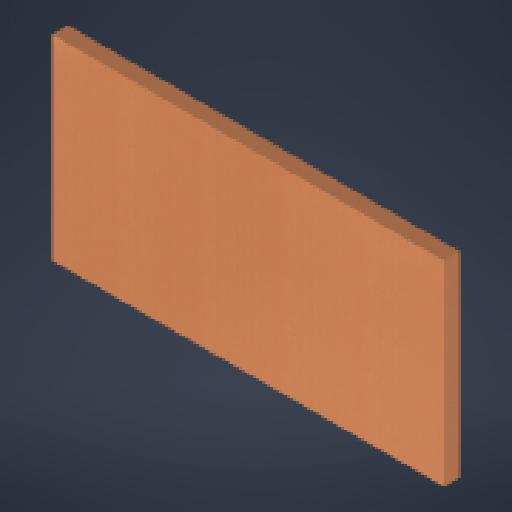
# Autodesk Inventor part: block_of_wood
Saved by Autodesk Inventor 2026 (Build 300175000, 175)
## iProperties
Created: 2025-03-30
Part Number: block_of_wood
Material: Wood (Walnut)
Document SubType Name: Modeling
Designer: paris
Density: 0.55 g/cm^3
Appearance: Walnut - Natural Polished
Author: paris
Autodesk Inventor part; units mm, degrees
ref_plane "YZ Plane" through (0, 0, 0) normal (1, 0, 0) x (0, 1, 0)
ref_plane "XZ Plane" through (0, 0, 0) normal (0, 1, 0) x (-1, 0, 0)
sketch "Sketch1" plane through (0, 0, 0) normal (0, 0, 1) x (1, 0, 0)
  line L0 (25, 1.485) -> (-25, 1.485) projected
  line L1 (0, 1.485) -> (-609.6, 1.485)
  line L2 (-609.6, 1.485) -> (-609.6, 611.085)
  line L3 (-609.6, 611.085) -> (0, 611.085)
  line L4 (0, 611.085) -> (0, 1.485)
  line L5 (0, 611.085) -> (609.6, 611.085)
  line L6 (609.6, 611.085) -> (609.6, 1.485)
  line L7 (609.6, 1.485) -> (0, 1.485)
  line L8 (0, 1.485) -> (0, 611.085)
  point P0 (0, 0)
  dimension "d0" = 609.6
  dimension "d1" = 609.6
  dimension "d2" = 609.6
  dimension "d3" = 609.6
  constraints: 16 end point, 4 parallel, 2 horizontal, 2 perpendicular, 1 midpoint
  measures "d0" distance of L2.end L3.end
  measures "d1" distance of L1.end L2.end
  measures "d2" distance of L6.end L7.end
  measures "d3" distance of L5.end L6.end
ref_plane "Work Plane1" through (-13.0355, 23.609, 49.4645) normal (0, 0, -1) x (0, 1, 0)
extrude "Extrusion1" add sketch "Sketch1" along normal up to surface (49.4645 mm away)
body "Solid1"
